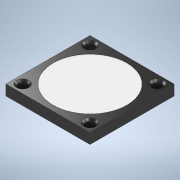
# Autodesk Inventor part: Filter
Saved by Autodesk Inventor 2020 (Build 240168000, 168)
## iProperties
Created: 2019-12-12
Part Number: Filter
Material: Generic
Document SubType Name: Modeling
Designer: nicoc
Density: 1 g/cm^3
Appearance: Glossy - Black
Author: nicoc
Autodesk Inventor part; units mm, degrees
ref_plane "YZ Plane" through (0, 0, 0) normal (1, 0, 0) x (0, 1, 0)
ref_plane "XZ Plane" through (0, 0, 0) normal (0, 1, 0) x (-1, 0, 0)
ref_plane "XY Plane" through (0, 0, 0) normal (0, 0, 1) x (1, 0, 0)
sketch "Sketch1" plane through (0, 0, 0) normal (0, 1, 0) x (-1, 0, 0)
  line L0 (0, 0) -> (40, 0)
  line L1 (40, 0) -> (40, -40)
  line L2 (40, -40) -> (0, -40)
  line L3 (0, -40) -> (0, 0)
  dimension "d0" = 40
  dimension "d1" = 40
  constraints: 8 end point, 2 parallel, 1 horizontal, 1 perpendicular
  measures "d0" distance between parallel lines of L2 L0
  measures "d1" distance between parallel lines of L1 L3
extrude "Extrusion1" add sketch "Sketch1" along normal blind 5
sketch "Sketch2" plane through (0, 5, 0) normal (0, 1, 0) x (1, 0, 0)
  line L0 (-40, 0) -> (0, 0) projected
  line L1 (0, 0) -> (0, 40) projected
  line L2 (0, 40) -> (-40, 40) projected
  line L3 (-40, 40) -> (-40, 0) projected
  point P0 (-4, 4)
  point P1 (-4, 36)
  point P2 (-36, 36)
  point P3 (-36, 4)
  dimension "d4" = 4
  dimension "d6" = 4
  dimension "d7" = 4
  dimension "d8" = 4
  dimension "d9" = 4
  dimension "d10" = 4
  dimension "d11" = 4
  dimension "d12" = 4
  measures "d4" distance from line of point (-4, 4) L0
  measures "d6" distance from line of point (-4, 4) L1
  measures "d7" distance from line of L1 point (-4, 36)
  measures "d8" distance from line of L2 point (-36, 36)
  measures "d9" distance from line of L3 point (-36, 36)
  measures "d10" distance from line of point (-36, 4) L0
  measures "d11" distance from line of L3 point (-36, 4)
  measures "d12" distance from line of point (-4, 36) L2
hole "Hole1" at (-4, 5, -4) at (-4, 5, -36) at (-36, 5, -36) at (-36, 5, -4) direction (0, -1, 0) diameter 4.3 end through all countersink diameter 6 countersink angle 90
sketch "Sketch3" plane through (0, 5, 0) normal (0, 1, 0) x (1, 0, 0)
  circle A0 centre (-20, 20) radius 17.5
  line L0 (-40, 0) -> (0, 0) projected
  line L1 (-40, 40) -> (-40, 0) projected
  dimension "d21" = 20
  dimension "d22" = 20
  dimension "d23" = 35
  constraints: 1 centre point
  measures "d21" distance from line of A0.centre L0
  measures "d22" distance from line of A0.centre L1
  measures "d23" diameter of A0
extrude "Extrusion2" cut sketch "Sketch3" against normal blind 0.1
equation "\"d4\" = d11"
equation "\"d6\" = d11"
equation "\"d7\" = d11"
equation "\"d8\" = d11"
equation "\"d9\" = d11"
equation "\"d10\" = d11"
equation "\"d12\" = d11"
body "Solid1"
